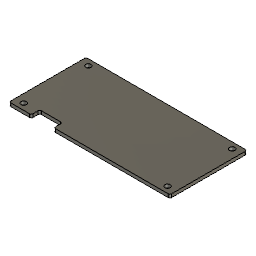
back_plate (Autodesk Fusion 360 design; units mm, degrees)
part number: 2025-12-15-21-34-38-126
Autodesk Fusion 360 part; units mm, degrees
sketch "Sketch1" plane through (0, 0, 0) normal (0, 0, 1) x (1, 0, 0)
  line L0 (0, 0) -> (96, 0)
  line L1 (96, 0) -> (96, 46)
  line L2 (96, 46) -> (0, 46)
  line L3 (0, 46) -> (0, 0)
  dimension "d1" = 96
  dimension "d2" = 46
  constraint horizontal L0
  constraint vertical L1
  constraint horizontal L2
  constraint vertical L3
  constraint coincident L0.start L3.end
  measures "d1" distance of L0.start L0.end
  measures "d2" distance of L0.start L2.end
extrude "Extrude1" add sketch "Sketch1" along normal blind 2
fillet "Fillet1" radius 1 4 edges at (96, 0, 1) (96, 46, 1) (0, 0, 1) (0, 46, 1)
sketch "Sketch2" plane through (0, 0, 2) normal (0, 0, 1) x (-1, 0, 0)
  arc A0 (-1, -46) -> (0, -45) centre (-1, -45) ccw
  line L0 (0, -45) -> (0, -1)
  arc A1 (0, -1) -> (-1, 0) centre (-1, -1) ccw
  line L1 (-1, 0) -> (-95, 0)
  arc A2 (-95, 0) -> (-96, -1) centre (-95, -1) ccw
  line L2 (-96, -1) -> (-96, -45)
  arc A3 (-96, -45) -> (-95, -46) centre (-95, -45) ccw
  line L3 (-95, -46) -> (-1, -46)
  line L4 (-13.3, 0) -> (-26.73, 0)
  line L5 (-26.73, 0) -> (-26.73, -4.065)
  line L6 (-25.73, -5.065) -> (-14.3, -5.065)
  line L7 (-13.3, -4.065) -> (-13.3, 0)
  arc A4 (-14.3, -5.065) -> (-13.3, -4.065) centre (-14.3, -4.065) ccw
  arc A5 (-26.73, -4.065) -> (-25.73, -5.065) centre (-25.73, -4.065) ccw
  point P0 (-13.3, -5.065)
  dimension "d7" = 13.43
  dimension "d8" = 5.065
  dimension "d9" = 13.3
  dimension "d10" = 5.065
  dimension "d11" = 1
  dimension "d12" = 1
  constraint horizontal L4
  constraint vertical L5
  constraint horizontal L6
  constraint vertical L7
  constraint coincident P0 L6
  constraint coincident P0 L7
  constraint tangent L6 A4
  constraint tangent L7 A4
  constraint tangent L5 A5
  constraint tangent L6 A5
  measures "d7" distance of L4.start L4.end
  measures "d8" distance of L4.start P0
  measures "d9" distance of L0 L7
  measures "d10" distance of L1 L6
  measures "d11" radius of A4
  measures "d12" radius of A5
extrude "Extrude2" cut sketch "Sketch2" against normal blind 2 contours L1 L4 L5 L6 L7 A4 A5
fillet "Fillet4" radius 1 2 edges at (13.3, 0, 1) (26.73, 0, 1)
sketch "Sketch5" plane through (0, 0, 2) normal (0, 0, 1) x (-1, 0, 0)
  arc A0 (-26.73, -1) -> (-27.73, 0) centre (-27.73, -1) ccw
  line L0 (-27.73, 0) -> (-95, 0)
  arc A1 (-95, 0) -> (-96, -1) centre (-95, -1) ccw
  line L1 (-96, -1) -> (-96, -45)
  arc A2 (-96, -45) -> (-95, -46) centre (-95, -45) ccw
  line L2 (-95, -46) -> (-1, -46)
  arc A3 (-1, -46) -> (0, -45) centre (-1, -45) ccw
  line L3 (0, -45) -> (0, -1)
  arc A4 (0, -1) -> (-1, 0) centre (-1, -1) ccw
  line L4 (-1, 0) -> (-12.3, 0)
  arc A5 (-12.3, 0) -> (-13.3, -1) centre (-12.3, -1) ccw
  line L5 (-13.3, -1) -> (-13.3, -4.065)
  arc A6 (-14.3, -5.065) -> (-13.3, -4.065) centre (-14.3, -4.065) ccw
  line L6 (-14.3, -5.065) -> (-25.73, -5.065)
  arc A7 (-26.73, -4.065) -> (-25.73, -5.065) centre (-25.73, -4.065) ccw
  line L7 (-26.73, -4.065) -> (-26.73, -1)
  circle A8 centre (-5.1, -3.75) radius 1.6
  circle A9 centre (-5.1, -42.25) radius 1.6
  circle A10 centre (-90.9, -3.75) radius 1.6
  circle A11 centre (-90.9, -42.25) radius 1.6
  dimension "d33" = 3.2
  dimension "d34" = 3.75
  dimension "d35" = 5.1
  dimension "d36" = 3.2
  dimension "d37" = 3.75
  dimension "d38" = 5.1
  dimension "d39" = 3.2
  dimension "d40" = 5.1
  dimension "d41" = 3.75
  dimension "d42" = 3.2
  dimension "d43" = 3.75
  dimension "d44" = 5.1
  measures "d33" diameter of A8
  measures "d34" distance of L4 A8.centre
  measures "d35" distance of L3 A8.centre
  measures "d36" diameter of A9
  measures "d37" distance of L2 A9.centre
  measures "d38" distance of L3 A9.centre
  measures "d39" diameter of A10
  measures "d40" distance of L1 A10.centre
  measures "d41" distance of L0 A10.centre
  measures "d42" diameter of A11
  measures "d43" distance of L2 A11.centre
  measures "d44" distance of L1 A11.centre
extrude "Extrude5" cut sketch "Sketch5" against normal blind 2 contours A8 | A9 | A10 | A11
equation "d8 = 4.69 mm - 0.375 mm + 0.75 mm"
equation "d10 = 4.69 mm - 0.375 mm + 0.75 mm"
